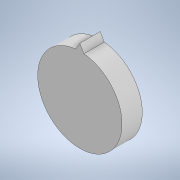
# Autodesk Inventor part: 12_ref
Saved by Autodesk Inventor 2021 (Build 250183000, 183)
## iProperties
Created: 2021-03-25
Part Number: 12_ref
Material: Generic
Document SubType Name: Modeling
Designer: lucia
Density: 1 g/cm^3
Appearance: Default
Author: lucia
Autodesk Inventor part; units mm, degrees
ref_plane "YZ Plane" through (0, 0, 0) normal (1, 0, 0) x (0, 1, 0)
ref_plane "XZ Plane" through (0, 0, 0) normal (0, 1, 0) x (-1, 0, 0)
ref_plane "XY Plane" through (0, 0, 0) normal (0, 0, 1) x (1, 0, 0)
sketch "Sketch1" plane through (0, 0, 0) normal (0, 0, 1) x (1, 0, 0)
  circle A0 centre (0, 0) radius 26.416
  line L0 (-2.54, 26.2936) -> (0, 30.693)
  line L1 (0, 30.693) -> (2.54, 26.2936)
  line L2 (-2.54, 26.2936) -> (2.54, 26.2936)
  dimension "d0" = 52.832
  dimension "d5" = 5.08
  constraints: 6 end point, 2 equal length, 2 point on circle, 1 centre point, 1 coincident, 1 horizontal
  measures "d0" diameter of A0
  measures "d5" distance of L0.start L1.end
extrude "Extrusion1" add sketch "Sketch1" against normal blind 12.7
equation "\"d0\" = 13.208 * scale"
equation "\"d5\" = 1.27 * scale"
equation "\"d1\" = 3.175 * scale"
equation "\"scale\" = 4"
body "Solid1"
